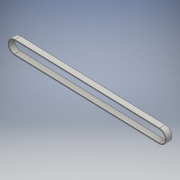
# Autodesk Inventor part: Tandrem
Saved by Autodesk Inventor 2016 (Build 200138000, 138)
## iProperties
Created: 2015-11-23
Part Number: Tandrem
Material: Generic
Document SubType Name: Modeling
Designer: iLyngklip
Density: 1 g/cm^3
Appearance: Default
Author: iLyngklip
Autodesk Inventor part; units mm, degrees
ref_plane "YZ Plane" through (0, 0, 0) normal (1, 0, 0) x (0, 1, 0)
ref_plane "XZ Plane" through (0, 0, 0) normal (0, 1, 0) x (-1, 0, 0)
ref_plane "Work Plane1" through (99.0561, 66.015, -1.0424) normal (0, 1, 0) x (-0.9985, 0, 0.0543)
sketch "Sketch1" plane through (99.0561, 66.015, -1.0424) normal (0, 1, 0) x (-0.9985, 0, 0.0543)
  circle A0 centre (-73.639, 4.9709) radius 7.75 projected
  arc A1 (-74.285, 11.1523) -> (-74.9346, 11.0494) centre (-73.639, 4.9709) ccw projected
  line L0 (-74.039, 10.5582) -> (-74.285, 11.1523) projected
  line L1 (-73.239, 10.5582) -> (-74.039, 10.5582) projected
  line L2 (-72.9929, 11.1523) -> (-73.239, 10.5582) projected
  arc A2 (-72.3433, 11.0494) -> (-72.9929, 11.1523) centre (-73.639, 4.9709) ccw projected
  line L3 (-72.2928, 10.4083) -> (-72.3433, 11.0494) projected
  line L4 (-71.532, 10.1611) -> (-72.2928, 10.4083) projected
  line L5 (-71.1144, 10.6501) -> (-71.532, 10.1611) projected
  arc A3 (-70.5284, 10.3515) -> (-71.1144, 10.6501) centre (-73.639, 4.9709) ccw projected
  line L6 (-70.6785, 9.7262) -> (-70.5284, 10.3515) projected
  line L7 (-70.0313, 9.256) -> (-70.6785, 9.7262) projected
  line L8 (-69.483, 9.592) -> (-70.0313, 9.256) projected
  arc A4 (-69.0179, 9.1269) -> (-69.483, 9.592) centre (-73.639, 4.9709) ccw projected
  line L9 (-69.3539, 8.5786) -> (-69.0179, 9.1269) projected
  line L10 (-68.8837, 7.9314) -> (-69.3539, 8.5786) projected
  line L11 (-68.2584, 8.0815) -> (-68.8837, 7.9314) projected
  arc A5 (-67.9598, 7.4955) -> (-68.2584, 8.0815) centre (-73.639, 4.9709) ccw projected
  line L12 (-68.4488, 7.0779) -> (-67.9598, 7.4955) projected
  line L13 (-68.2016, 6.3171) -> (-68.4488, 7.0779) projected
  line L14 (-67.5605, 6.2666) -> (-68.2016, 6.3171) projected
  arc A6 (-67.4576, 5.617) -> (-67.5605, 6.2666) centre (-73.639, 4.9709) ccw projected
  line L15 (-68.0517, 5.3709) -> (-67.4576, 5.617) projected
  line L16 (-68.0517, 4.5709) -> (-68.0517, 5.3709) projected
  line L17 (-67.4576, 4.3249) -> (-68.0517, 4.5709) projected
  arc A7 (-67.5605, 3.6753) -> (-67.4576, 4.3249) centre (-73.639, 4.9709) ccw projected
  line L18 (-68.2016, 3.6248) -> (-67.5605, 3.6753) projected
  line L19 (-68.4488, 2.864) -> (-68.2016, 3.6248) projected
  line L20 (-67.9598, 2.4463) -> (-68.4488, 2.864) projected
  arc A8 (-68.2584, 1.8603) -> (-67.9598, 2.4463) centre (-73.639, 4.9709) ccw projected
  line L21 (-68.8837, 2.0105) -> (-68.2584, 1.8603) projected
  line L22 (-69.3539, 1.3632) -> (-68.8837, 2.0105) projected
  line L23 (-69.0179, 0.815) -> (-69.3539, 1.3632) projected
  arc A9 (-69.483, 0.3499) -> (-69.0179, 0.815) centre (-73.639, 4.9709) ccw projected
  line L24 (-70.0313, 0.6859) -> (-69.483, 0.3499) projected
  line L25 (-70.6785, 0.2157) -> (-70.0313, 0.6859) projected
  line L26 (-70.5284, -0.4096) -> (-70.6785, 0.2157) projected
  arc A10 (-71.1144, -0.7082) -> (-70.5284, -0.4096) centre (-73.639, 4.9709) ccw projected
  line L27 (-71.532, -0.2192) -> (-71.1144, -0.7082) projected
  line L28 (-72.2928, -0.4664) -> (-71.532, -0.2192) projected
  line L29 (-72.3433, -1.1075) -> (-72.2928, -0.4664) projected
  arc A11 (-72.9929, -1.2104) -> (-72.3433, -1.1075) centre (-73.639, 4.9709) ccw projected
  line L30 (-73.239, -0.6163) -> (-72.9929, -1.2104) projected
  line L31 (-74.039, -0.6163) -> (-73.239, -0.6163) projected
  line L32 (-74.285, -1.2104) -> (-74.039, -0.6163) projected
  arc A12 (-74.9346, -1.1075) -> (-74.285, -1.2104) centre (-73.639, 4.9709) ccw projected
  line L33 (-74.9851, -0.4664) -> (-74.9346, -1.1075) projected
  line L34 (-75.7459, -0.2192) -> (-74.9851, -0.4664) projected
  line L35 (-76.1636, -0.7082) -> (-75.7459, -0.2192) projected
  arc A13 (-76.7496, -0.4096) -> (-76.1636, -0.7082) centre (-73.639, 4.9709) ccw projected
  line L36 (-76.5994, 0.2157) -> (-76.7496, -0.4096) projected
  line L37 (-77.2467, 0.6859) -> (-76.5994, 0.2157) projected
  line L38 (-77.7949, 0.3499) -> (-77.2467, 0.6859) projected
  arc A14 (-78.26, 0.815) -> (-77.7949, 0.3499) centre (-73.639, 4.9709) ccw projected
  line L39 (-77.924, 1.3632) -> (-78.26, 0.815) projected
  line L40 (-78.3942, 2.0105) -> (-77.924, 1.3632) projected
  line L41 (-79.0195, 1.8603) -> (-78.3942, 2.0105) projected
  arc A15 (-79.3181, 2.4463) -> (-79.0195, 1.8603) centre (-73.639, 4.9709) ccw projected
  line L42 (-78.8291, 2.864) -> (-79.3181, 2.4463) projected
  line L43 (-79.0763, 3.6248) -> (-78.8291, 2.864) projected
  line L44 (-79.7174, 3.6753) -> (-79.0763, 3.6248) projected
  arc A16 (-79.8203, 4.3249) -> (-79.7174, 3.6753) centre (-73.639, 4.9709) ccw projected
  line L45 (-79.2262, 4.5709) -> (-79.8203, 4.3249) projected
  line L46 (-79.2262, 5.3709) -> (-79.2262, 4.5709) projected
  line L47 (-79.8203, 5.617) -> (-79.2262, 5.3709) projected
  arc A17 (-79.7174, 6.2666) -> (-79.8203, 5.617) centre (-73.639, 4.9709) ccw projected
  line L48 (-79.0763, 6.3171) -> (-79.7174, 6.2666) projected
  line L49 (-78.8291, 7.0779) -> (-79.0763, 6.3171) projected
  line L50 (-79.3181, 7.4955) -> (-78.8291, 7.0779) projected
  arc A18 (-79.0195, 8.0815) -> (-79.3181, 7.4955) centre (-73.639, 4.9709) ccw projected
  line L51 (-78.3942, 7.9314) -> (-79.0195, 8.0815) projected
  line L52 (-77.924, 8.5786) -> (-78.3942, 7.9314) projected
  line L53 (-78.26, 9.1269) -> (-77.924, 8.5786) projected
  arc A19 (-77.7949, 9.592) -> (-78.26, 9.1269) centre (-73.639, 4.9709) ccw projected
  line L54 (-77.2467, 9.256) -> (-77.7949, 9.592) projected
  line L55 (-76.5994, 9.7262) -> (-77.2467, 9.256) projected
  line L56 (-76.7496, 10.3515) -> (-76.5994, 9.7262) projected
  arc A20 (-76.1636, 10.6501) -> (-76.7496, 10.3515) centre (-73.639, 4.9709) ccw projected
  line L57 (-75.7459, 10.1611) -> (-76.1636, 10.6501) projected
  line L58 (-74.9851, 10.4083) -> (-75.7459, 10.1611) projected
  line L59 (-74.9346, 11.0494) -> (-74.9851, 10.4083) projected
  circle A21 centre (76.3213, 1.5167) radius 8.5 projected
  arc A22 (76.017, 7.7243) -> (75.3526, 7.6558) centre (76.3213, 1.5167) ccw projected
  line L60 (76.226, 7.1302) -> (76.017, 7.7243) projected
  line L61 (77.0249, 7.0867) -> (76.226, 7.1302) projected
  line L62 (77.2971, 7.6546) -> (77.0249, 7.0867) projected
  arc A23 (77.9501, 7.5145) -> (77.2971, 7.6546) centre (76.3213, 1.5167) ccw projected
  line L63 (77.9654, 6.8849) -> (77.9501, 7.5145) projected
  line L64 (78.7116, 6.5967) -> (77.9654, 6.8849) projected
  line L65 (79.1461, 7.0527) -> (78.7116, 6.5967) projected
  arc A24 (79.7238, 6.7176) -> (79.1461, 7.0527) centre (76.3213, 1.5167) ccw projected
  line L66 (79.5437, 6.1141) -> (79.7238, 6.7176) projected
  line L67 (80.1645, 5.6094) -> (79.5437, 6.1141) projected
  line L68 (80.7185, 5.9088) -> (80.1645, 5.6094) projected
  arc A25 (81.1644, 5.4116) -> (80.7185, 5.9088) centre (76.3213, 1.5167) ccw projected
  line L69 (80.8067, 4.8933) -> (81.1644, 5.4116) projected
  line L70 (81.2411, 4.2215) -> (80.8067, 4.8933) projected
  line L71 (81.8605, 4.335) -> (81.2411, 4.2215) projected
  arc A26 (82.131, 3.7243) -> (81.8605, 4.335) centre (76.3213, 1.5167) ccw projected
  line L72 (81.6306, 3.3419) -> (82.131, 3.7243) projected
  line L73 (81.8361, 2.5688) -> (81.6306, 3.3419) projected
  line L74 (82.4603, 2.4853) -> (81.8361, 2.5688) projected
  arc A27 (82.5288, 1.821) -> (82.4603, 2.4853) centre (76.3213, 1.5167) ccw projected
  line L75 (81.9347, 1.6119) -> (82.5288, 1.821) projected
  line L76 (81.8913, 0.8131) -> (81.9347, 1.6119) projected
  line L77 (82.4592, 0.5409) -> (81.8913, 0.8131) projected
  arc A28 (82.319, -0.1121) -> (82.4592, 0.5409) centre (76.3213, 1.5167) ccw projected
  line L78 (81.6894, -0.1274) -> (82.319, -0.1121) projected
  line L79 (81.4012, -0.8737) -> (81.6894, -0.1274) projected
  line L80 (81.8572, -1.3081) -> (81.4012, -0.8737) projected
  arc A29 (81.5221, -1.8858) -> (81.8572, -1.3081) centre (76.3213, 1.5167) ccw projected
  line L81 (80.9186, -1.7058) -> (81.5221, -1.8858) projected
  line L82 (80.4139, -2.3265) -> (80.9186, -1.7058) projected
  line L83 (80.7133, -2.8805) -> (80.4139, -2.3265) projected
  arc A30 (80.2161, -3.3264) -> (80.7133, -2.8805) centre (76.3213, 1.5167) ccw projected
  line L84 (79.6978, -2.9687) -> (80.2161, -3.3264) projected
  line L85 (79.026, -3.4031) -> (79.6978, -2.9687) projected
  line L86 (79.1395, -4.0225) -> (79.026, -3.4031) projected
  arc A31 (78.5289, -4.293) -> (79.1395, -4.0225) centre (76.3213, 1.5167) ccw projected
  line L87 (78.1465, -3.7926) -> (78.5289, -4.293) projected
  line L88 (77.3733, -3.9981) -> (78.1465, -3.7926) projected
  line L89 (77.2899, -4.6223) -> (77.3733, -3.9981) projected
  arc A32 (76.6255, -4.6908) -> (77.2899, -4.6223) centre (76.3213, 1.5167) ccw projected
  line L90 (76.4165, -4.0967) -> (76.6255, -4.6908) projected
  line L91 (75.6177, -4.0533) -> (76.4165, -4.0967) projected
  line L92 (75.3454, -4.6212) -> (75.6177, -4.0533) projected
  arc A33 (74.6924, -4.481) -> (75.3454, -4.6212) centre (76.3213, 1.5167) ccw projected
  line L93 (74.6772, -3.8514) -> (74.6924, -4.481) projected
  line L94 (73.9309, -3.5632) -> (74.6772, -3.8514) projected
  line L95 (73.4964, -4.0192) -> (73.9309, -3.5632) projected
  arc A34 (72.9187, -3.6841) -> (73.4964, -4.0192) centre (76.3213, 1.5167) ccw projected
  line L96 (73.0988, -3.0806) -> (72.9187, -3.6841) projected
  line L97 (72.4781, -2.5759) -> (73.0988, -3.0806) projected
  line L98 (71.924, -2.8754) -> (72.4781, -2.5759) projected
  arc A35 (71.4781, -2.3781) -> (71.924, -2.8754) centre (76.3213, 1.5167) ccw projected
  line L99 (71.8358, -1.8598) -> (71.4781, -2.3781) projected
  line L100 (71.4015, -1.188) -> (71.8358, -1.8598) projected
  line L101 (70.782, -1.3016) -> (71.4015, -1.188) projected
  arc A36 (70.5116, -0.6909) -> (70.782, -1.3016) centre (76.3213, 1.5167) ccw projected
  line L102 (71.012, -0.3085) -> (70.5116, -0.6909) projected
  line L103 (70.8064, 0.4647) -> (71.012, -0.3085) projected
  line L104 (70.1822, 0.5481) -> (70.8064, 0.4647) projected
  arc A37 (70.1137, 1.2125) -> (70.1822, 0.5481) centre (76.3213, 1.5167) ccw projected
  line L105 (70.7078, 1.4215) -> (70.1137, 1.2125) projected
  line L106 (70.7513, 2.2203) -> (70.7078, 1.4215) projected
  line L107 (70.1834, 2.4926) -> (70.7513, 2.2203) projected
  arc A38 (70.3235, 3.1456) -> (70.1834, 2.4926) centre (76.3213, 1.5167) ccw projected
  line L108 (70.9531, 3.1608) -> (70.3235, 3.1456) projected
  line L109 (71.2413, 3.9071) -> (70.9531, 3.1608) projected
  line L110 (70.7853, 4.3415) -> (71.2413, 3.9071) projected
  arc A39 (71.1204, 4.9193) -> (70.7853, 4.3415) centre (76.3213, 1.5167) ccw projected
  line L111 (71.7239, 4.7392) -> (71.1204, 4.9193) projected
  line L112 (72.2286, 5.3599) -> (71.7239, 4.7392) projected
  line L113 (71.9292, 5.914) -> (72.2286, 5.3599) projected
  arc A40 (72.4264, 6.3599) -> (71.9292, 5.914) centre (76.3213, 1.5167) ccw projected
  line L114 (72.9447, 6.0021) -> (72.4264, 6.3599) projected
  line L115 (73.6165, 6.4365) -> (72.9447, 6.0021) projected
  line L116 (73.503, 7.056) -> (73.6165, 6.4365) projected
  arc A41 (74.1136, 7.3264) -> (73.503, 7.056) centre (76.3213, 1.5167) ccw projected
  line L117 (74.496, 6.826) -> (74.1136, 7.3264) projected
  line L118 (75.2692, 7.0315) -> (74.496, 6.826) projected
  line L119 (75.3526, 7.6558) -> (75.2692, 7.0315) projected
  line L120 (76.1551, -5.6964) -> (-73.8051, -2.2421)
  line L121 (76.4874, 8.7298) -> (-73.4728, 12.184)
  arc A42 (76.1551, -5.6964) -> (76.4874, 8.7298) centre (76.3213, 1.5167) ccw
  arc A43 (-73.4958, 11.1843) -> (-73.7821, -1.2424) centre (-73.639, 4.9709) ccw
  arc A44 (-73.4728, 12.184) -> (-73.8051, -2.2421) centre (-73.639, 4.9709) ccw
  line L122 (-73.7821, -1.2424) -> (76.1781, -4.6966)
  arc A45 (76.1781, -4.6966) -> (76.017, 7.7243) centre (76.3213, 1.5167) ccw
  line L123 (76.4644, 7.7301) -> (-73.4958, 11.1843)
  point P0 (98.9665, -4.3398)
  dimension "d1" = 1
  dimension "d2" = 1
  constraints: 16 end point, 11 point on circle, 8 tangent, 4 centre point, 4 coincident, 1 point on line
  measures "d1" radial gap between concentric circles of A44 A43
  measures "d2" radial gap between concentric circles of A42 A45
extrude "Extrusion1" add sketch "Sketch1" along normal blind 6 contours L123 A43 A1 A20 A19 A18 A17 A16 A15 A14 A13 A12 L122 A0 L120 A44 L121 | A0 L121 A21 L123 | L122 A21 L120 A0 | A21 L121 A42 L120 L122 A45 A32 A31 A30 A29 A28 A27 A26 A25 A24 A23 L123
body "Solid1"
